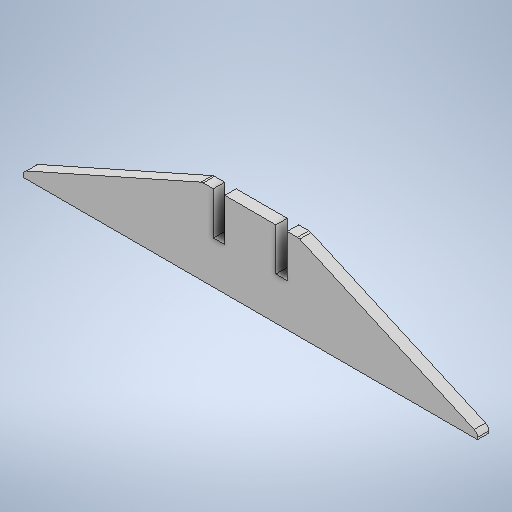
# Autodesk Inventor part: LegLessMaterial
Saved by Autodesk Inventor 2025.1 (Build 291241000, 241)
## iProperties
Created: 2025-03-30
Part Number: LegLessMaterial
Material: Všeobecné
Document SubType Name: Modeling
Designer: 42060
Density: 1 g/cm^3
Appearance: Výchozí
Author: 42060
Autodesk Inventor part; units mm, degrees
ref_plane "YZ Plane" through (0, 0, 0) normal (1, 0, 0) x (0, 1, 0)
ref_plane "XZ Plane" through (0, 0, 0) normal (0, 1, 0) x (-1, 0, 0)
ref_plane "XY Plane" through (0, 0, 0) normal (0, 0, 1) x (1, 0, 0)
sketch "Náčrt1" plane through (0, 0, 0) normal (0, 0, 1) x (1, 0, 0)
  line L0 (0, 0) -> (0, 30)
  line L1 (0, 30) -> (-9, 30)
  line L2 (-9, 30) -> (-9, 15)
  line L3 (-9, 15) -> (-13, 15)
  line L4 (-13, 15) -> (-13, 30)
  line L5 (-13, 30) -> (-16.5756, 30)
  line L6 (-17.3878, 29.8276) -> (-78.8123, 2.5279)
  line L7 (-80, 0.7003) -> (-80, 0)
  line L8 (-80, 0) -> (0, 0)
  arc A0 (-78.8123, 2.5279) -> (-80, 0.7003) centre (-78, 0.7003) ccw
  arc A1 (-16.5756, 30) -> (-17.3878, 29.8276) centre (-16.5756, 28) ccw
  line L9 (0, 30) -> (9, 30)
  line L10 (9, 30) -> (9, 15)
  line L11 (9, 15) -> (13, 15)
  line L12 (13, 15) -> (13, 30)
  line L13 (13, 30) -> (16.5756, 30)
  line L14 (17.3878, 29.8276) -> (78.8123, 2.5279)
  line L15 (80, 0.7003) -> (80, 0)
  line L16 (80, 0) -> (0, 0)
  arc A2 (80, 0.7003) -> (78.8123, 2.5279) centre (78, 0.7003) ccw
  arc A3 (17.3878, 29.8276) -> (16.5756, 30) centre (16.5756, 28) ccw
  point P0 (-17, 30)
  point P1 (-80, 2)
  point P2 (17, 30)
  point P3 (80, 2)
  dimension "d0" = 15
  dimension "d1" = 15
  dimension "d4" = 4
  dimension "d5" = 4
  dimension "d6" = 9
  dimension "d7" = 2
  dimension "d8" = 80
  dimension "d9" = 2
  constraints: 34 end point, 13 symmetric about line, 12 point on line, 8 point on circle, 5 perpendicular, 4 centre point, 4 tangent, 2 vertical, 1 equal radius, 2 other
  measures "d0" distance between parallel lines of L1 L3
  measures "d1" distance between parallel lines of L8 L3
  measures "d4" distance between parallel lines of L2 L4
  measures "d5" distance of L4.end point (-17, 30)
  measures "d6" distance between parallel lines of L0 L2
  measures "d7" distance of point (-80, 2) L7.end
  measures "d8" distance between parallel lines of L7 L0
  measures "d9" radius of A0
extrude "Vysunutí1" add sketch "Náčrt1" along normal mid plane 4
equation "\"d10\" = d4"
